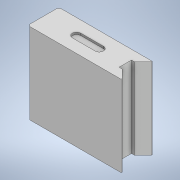
# Autodesk Inventor part: Призма-5
Saved by Autodesk Inventor 2022 (Build 260153000, 153)
## iProperties
Created: 2021-12-03
Part Number: Призма-5
Material: Типовые
Document SubType Name: Modeling
Designer: Украинцев
Density: 1 g/cm^3
Appearance: По умолчанию
Author: Украинцев
Autodesk Inventor part; units mm, degrees
ref_plane "YZ Plane" through (0, 0, 0) normal (1, 0, 0) x (0, 1, 0)
ref_plane "XZ Plane" through (0, 0, 0) normal (0, 1, 0) x (-1, 0, 0)
ref_plane "XY Plane" through (0, 0, 0) normal (0, 0, 1) x (1, 0, 0)
sketch "Эскиз1" plane through (0, 0, 0) normal (0, 1, 0) x (-1, 0, 0)
  line L0 (45, 15) -> (-45, 15)
  line L1 (-45, 15) -> (-45, -15)
  line L2 (-45, -15) -> (45, -15)
  line L3 (45, -15) -> (45, 15)
  line L4 (45, 15) -> (-45, -15) construction
  line L5 (-45, 15) -> (45, -15) construction
  line L6 (-45, 15) -> (-9, 15)
  line L7 (-9, 15) -> (-9, 0)
  line L8 (-9, 0) -> (13, 0)
  line L9 (13, 0) -> (-9, 0) construction
  line L10 (-45, -15) -> (-34, -15)
  line L11 (-34, -15) -> (-34, 0)
  line L12 (-34, 0) -> (-34, -6)
  line L13 (-45, -15) -> (-45, -14)
  line L14 (-45, 15) -> (-45, 14)
  line L15 (-45, -14) -> (-28.0294, -14) construction
  line L16 (-34, -6) -> (-37, -6)
  line L17 (-34, 0) -> (-34, 6)
  line L18 (-34, 6) -> (-37, 6)
  line L19 (-37, 6) -> (-45, 14)
  line L20 (-45, -14) -> (-37, -6)
  line L21 (-45, 0) -> (-51.506, 0)
  circle A0 centre (-51, 0) radius 14.1421
  line L22 (-9, 0) -> (13, 0) construction
  line L23 (-9, -4) -> (13, -4)
  line L24 (13, 4) -> (-9, 4)
  arc A1 (-9, 4) -> (-9, -4) centre (-9, 0) ccw
  arc A2 (13, -4) -> (13, 4) centre (13, 0) ccw
  point P0 (0, 0)
  point P1 (2, 0)
  point P2 (2, 0)
  dimension "d0" = 90
  dimension "d1" = 30
  dimension "d2" = 36
  dimension "d3" = 22
  dimension "d7" = 11
  dimension "d8" = 6
  dimension "d9" = 1
  dimension "d10" = 1
  dimension "d12" = 6
  dimension "d13" = 3
  dimension "d14" = 6.506
  dimension "d17" = 8
  constraints: 54 end point, 6 horizontal, 6 point on line, 5 midpoint, 5 perpendicular, 4 point on circle, 4 tangent, 3 centre point, 3 parallel, 1 vertical
  measures "d0" distance of L2.end L1.end
  measures "d1" distance of L1.end L0.end
  measures "d2" distance of L0.end L6.end
  measures "d3" distance of L7.end L8.end
  measures "d7" distance of L1.end L10.end
  measures "d8" distance of L11.end L12.end
  measures "d9" distance of L1.end L13.end
  measures "d10" distance of L0.end L14.end
  measures "d12" distance of L11.end L17.end
  measures "d13" distance of L17.end L18.end
  measures "d14" distance of L21.start L21.end
  measures "d17" diameter of A2
extrude "Выдавливание1" add sketch "Эскиз1" along normal blind 39 contours L3 L2 L11 L17 L18 L19 L1 L0 | L2 L1 L20 L16 L11 | A1 L24 A2 L23
extrude "Выдавливание2" cut sketch "Эскиз1" along normal blind 2 contours A1 L24 A2 L23
mirror "Зеркальное отражение1" about plane through (0, 39, 0) normal (0, 1, 0) of "Выдавливание2", "Выдавливание1"
chamfer "Фаска1" distance 2 angle 45 2 edges at (-45, 39, -15) (-45, 39, 15)
